Autodesk Fusion 360 part; units mm, degrees
(part 27 of 40)
  spline S73 degree 5 poles (31.1115, 52.5103) (31.1272, 52.5368) (31.1594, 52.5895) (31.2097, 52.6672) (31.2807, 52.7681) (31.3748, 52.8906) (31.4727, 53.0106) (31.5729, 53.1289) (31.6744, 53.2464) (31.7767, 53.3634) (31.88, 53.4797) (31.9844, 53.5951) (32.0903, 53.7094) (32.1981, 53.8224) (32.3077, 53.934) (32.419, 54.0444) (32.5316, 54.1537) (32.6455, 54.2622) (32.7603, 54.3698) (32.876, 54.4767) (32.9927, 54.5828) (33.1105, 54.6881) (33.2292, 54.7926) (33.3491, 54.8961) (33.47, 54.9988) (33.5919, 55.1007) (33.7148, 55.2017) (33.8386, 55.302) (33.9633, 55.4015) (34.0888, 55.5003) (34.2151, 55.5984) (34.3423, 55.6957) (34.4703, 55.7923) (34.5991, 55.8881) (34.7288, 55.9832) (34.8592, 56.0776) (34.9905, 56.1712) (35.1224, 56.2642) (35.2552, 56.3564) (35.3886, 56.448) (35.5228, 56.5388) (35.6577, 56.629) (35.7933, 56.7185) (35.9295, 56.8073) (36.0665, 56.8955) (36.2042, 56.9829) (36.3425, 57.0697) (36.4815, 57.1558) (36.6211, 57.2413) (36.7614, 57.3261) (36.9023, 57.4102) (37.0438, 57.4937) (37.186, 57.5765) (37.3288, 57.6587) (37.4721, 57.7403) (37.6161, 57.8212) (37.7607, 57.9014) (37.9058, 57.981) (38.0515, 58.06) (38.1978, 58.1383) (38.3447, 58.216) (38.4921, 58.2931) (38.6401, 58.3695) (38.7886, 58.4453) (38.9377, 58.5205) (39.0873, 58.595) (39.2374, 58.669) (39.3881, 58.7423) (39.5393, 58.8149) (39.6909, 58.887) (39.8431, 58.9584) (39.9653, 59.0151) (40.0572, 59.0573) (40.1185, 59.0853) (40.1492, 59.0993) knots 0 0 0 0 0 0 0.01428571 0.02857143 0.04285714 0.05714286 0.07142857 0.08571429 0.1 0.11428571 0.12857143 0.14285714 0.15714286 0.17142857 0.18571429 0.2 0.21428571 0.22857143 0.24285714 0.25714286 0.27142857 0.28571429 0.3 0.31428571 0.32857143 0.34285714 0.35714286 0.37142857 0.38571429 0.4 0.41428571 0.42857143 0.44285714 0.45714286 0.47142857 0.48571429 0.5 0.51428571 0.52857143 0.54285714 0.55714286 0.57142857 0.58571429 0.6 0.61428571 0.62857143 0.64285714 0.65714286 0.67142857 0.68571429 0.7 0.71428571 0.72857143 0.74285714 0.75714286 0.77142857 0.78571429 0.8 0.81428571 0.82857143 0.84285714 0.85714286 0.87142857 0.88571429 0.9 0.91428571 0.92857143 0.94285714 0.95714286 0.97142857 0.98571429 1 1 1 1 1 1
  line L5468 (31.1115, 52.5103) -> (31.1272, 52.5368) construction
  line L5469 (31.1272, 52.5368) -> (31.1594, 52.5895) construction
  line L5470 (31.1594, 52.5895) -> (31.2097, 52.6672) construction
  line L5471 (31.2097, 52.6672) -> (31.2807, 52.7681) construction
  line L5472 (31.2807, 52.7681) -> (31.3748, 52.8906) construction
  line L5473 (31.3748, 52.8906) -> (31.4727, 53.0106) construction
  line L5474 (31.4727, 53.0106) -> (31.5729, 53.1289) construction
  line L5475 (31.5729, 53.1289) -> (31.6744, 53.2464) construction
  line L5476 (31.6744, 53.2464) -> (31.7767, 53.3634) construction
  line L5477 (31.7767, 53.3634) -> (31.88, 53.4797) construction
  line L5478 (31.88, 53.4797) -> (31.9844, 53.5951) construction
  line L5479 (31.9844, 53.5951) -> (32.0903, 53.7094) construction
  line L5480 (32.0903, 53.7094) -> (32.1981, 53.8224) construction
  line L5481 (32.1981, 53.8224) -> (32.3077, 53.934) construction
  line L5482 (32.3077, 53.934) -> (32.419, 54.0444) construction
  line L5483 (32.419, 54.0444) -> (32.5316, 54.1537) construction
  line L5484 (32.5316, 54.1537) -> (32.6455, 54.2622) construction
  line L5485 (32.6455, 54.2622) -> (32.7603, 54.3698) construction
  line L5486 (32.7603, 54.3698) -> (32.876, 54.4767) construction
  line L5487 (32.876, 54.4767) -> (32.9927, 54.5828) construction
  line L5488 (32.9927, 54.5828) -> (33.1105, 54.6881) construction
  line L5489 (33.1105, 54.6881) -> (33.2292, 54.7926) construction
  line L5490 (33.2292, 54.7926) -> (33.3491, 54.8961) construction
  line L5491 (33.3491, 54.8961) -> (33.47, 54.9988) construction
  line L5492 (33.47, 54.9988) -> (33.5919, 55.1007) construction
  line L5493 (33.5919, 55.1007) -> (33.7148, 55.2017) construction
  line L5494 (33.7148, 55.2017) -> (33.8386, 55.302) construction
  line L5495 (33.8386, 55.302) -> (33.9633, 55.4015) construction
  line L5496 (33.9633, 55.4015) -> (34.0888, 55.5003) construction
  line L5497 (34.0888, 55.5003) -> (34.2151, 55.5984) construction
  line L5498 (34.2151, 55.5984) -> (34.3423, 55.6957) construction
  line L5499 (34.3423, 55.6957) -> (34.4703, 55.7923) construction
  line L5500 (34.4703, 55.7923) -> (34.5991, 55.8881) construction
  line L5501 (34.5991, 55.8881) -> (34.7288, 55.9832) construction
  line L5502 (34.7288, 55.9832) -> (34.8592, 56.0776) construction
  line L5503 (34.8592, 56.0776) -> (34.9905, 56.1712) construction
  line L5504 (34.9905, 56.1712) -> (35.1224, 56.2642) construction
  line L5505 (35.1224, 56.2642) -> (35.2552, 56.3564) construction
  line L5506 (35.2552, 56.3564) -> (35.3886, 56.448) construction
  line L5507 (35.3886, 56.448) -> (35.5228, 56.5388) construction
  line L5508 (35.5228, 56.5388) -> (35.6577, 56.629) construction
  line L5509 (35.6577, 56.629) -> (35.7933, 56.7185) construction
  line L5510 (35.7933, 56.7185) -> (35.9295, 56.8073) construction
  line L5511 (35.9295, 56.8073) -> (36.0665, 56.8955) construction
  line L5512 (36.0665, 56.8955) -> (36.2042, 56.9829) construction
  line L5513 (36.2042, 56.9829) -> (36.3425, 57.0697) construction
  line L5514 (36.3425, 57.0697) -> (36.4815, 57.1558) construction
  line L5515 (36.4815, 57.1558) -> (36.6211, 57.2413) construction
  line L5516 (36.6211, 57.2413) -> (36.7614, 57.3261) construction
  line L5517 (36.7614, 57.3261) -> (36.9023, 57.4102) construction
  line L5518 (36.9023, 57.4102) -> (37.0438, 57.4937) construction
  line L5519 (37.0438, 57.4937) -> (37.186, 57.5765) construction
  line L5520 (37.186, 57.5765) -> (37.3288, 57.6587) construction
  line L5521 (37.3288, 57.6587) -> (37.4721, 57.7403) construction
  line L5522 (37.4721, 57.7403) -> (37.6161, 57.8212) construction
  line L5523 (37.6161, 57.8212) -> (37.7607, 57.9014) construction
  line L5524 (37.7607, 57.9014) -> (37.9058, 57.981) construction
  line L5525 (37.9058, 57.981) -> (38.0515, 58.06) construction
  line L5526 (38.0515, 58.06) -> (38.1978, 58.1383) construction
  line L5527 (38.1978, 58.1383) -> (38.3447, 58.216) construction
  line L5528 (38.3447, 58.216) -> (38.4921, 58.2931) construction
  line L5529 (38.4921, 58.2931) -> (38.6401, 58.3695) construction
  line L5530 (38.6401, 58.3695) -> (38.7886, 58.4453) construction
  line L5531 (38.7886, 58.4453) -> (38.9377, 58.5205) construction
  line L5532 (38.9377, 58.5205) -> (39.0873, 58.595) construction
  line L5533 (39.0873, 58.595) -> (39.2374, 58.669) construction
  line L5534 (39.2374, 58.669) -> (39.3881, 58.7423) construction
  line L5535 (39.3881, 58.7423) -> (39.5393, 58.8149) construction
  line L5536 (39.5393, 58.8149) -> (39.6909, 58.887) construction
  line L5537 (39.6909, 58.887) -> (39.8431, 58.9584) construction
  line L5538 (39.8431, 58.9584) -> (39.9653, 59.0151) construction
  line L5539 (39.9653, 59.0151) -> (40.0572, 59.0573) construction
  line L5540 (40.0572, 59.0573) -> (40.1185, 59.0853) construction
  line L5541 (40.1185, 59.0853) -> (40.1492, 59.0993) construction
  arc A139 (51.9354, 24.5301) -> (54.5366, 23.5481) centre (53.7438, 25.3842) ccw
  spline S74 degree 5 poles (52.5103, -31.1115) (52.5368, -31.1272) (52.5895, -31.1594) (52.6672, -31.2097) (52.7681, -31.2807) (52.8906, -31.3748) (53.0106, -31.4727) (53.1289, -31.5729) (53.2464, -31.6744) (53.3634, -31.7767) (53.4797, -31.88) (53.5951, -31.9844) (53.7094, -32.0903) (53.8224, -32.1981) (53.934, -32.3077) (54.0444, -32.419) (54.1537, -32.5316) (54.2622, -32.6455) (54.3698, -32.7603) (54.4767, -32.876) (54.5828, -32.9927) (54.6881, -33.1105) (54.7926, -33.2292) (54.8961, -33.3491) (54.9988, -33.47) (55.1007, -33.5919) (55.2017, -33.7148) (55.302, -33.8386) (55.4015, -33.9633) (55.5003, -34.0888) (55.5984, -34.2151) (55.6957, -34.3423) (55.7923, -34.4703) (55.8881, -34.5991) (55.9832, -34.7288) (56.0776, -34.8592) (56.1712, -34.9905) (56.2642, -35.1224) (56.3564, -35.2552) (56.448, -35.3886) (56.5388, -35.5228) (56.629, -35.6577) (56.7185, -35.7933) (56.8073, -35.9295) (56.8955, -36.0665) (56.9829, -36.2042) (57.0697, -36.3425) (57.1558, -36.4815) (57.2413, -36.6211) (57.3261, -36.7614) (57.4102, -36.9023) (57.4937, -37.0438) (57.5765, -37.186) (57.6587, -37.3288) (57.7403, -37.4721) (57.8212, -37.6161) (57.9014, -37.7607) (57.981, -37.9058) (58.06, -38.0515) (58.1383, -38.1978) (58.216, -38.3447) (58.2931, -38.4921) (58.3695, -38.6401) (58.4453, -38.7886) (58.5205, -38.9377) (58.595, -39.0873) (58.669, -39.2374) (58.7423, -39.3881) (58.8149, -39.5393) (58.887, -39.6909) (58.9584, -39.8431) (59.0151, -39.9653) (59.0573, -40.0572) (59.0853, -40.1185) (59.0993, -40.1492) knots 0 0 0 0 0 0 0.01428571 0.02857143 0.04285714 0.05714286 0.07142857 0.08571429 0.1 0.11428571 0.12857143 0.14285714 0.15714286 0.17142857 0.18571429 0.2 0.21428571 0.22857143 0.24285714 0.25714286 0.27142857 0.28571429 0.3 0.31428571 0.32857143 0.34285714 0.35714286 0.37142857 0.38571429 0.4 0.41428571 0.42857143 0.44285714 0.45714286 0.47142857 0.48571429 0.5 0.51428571 0.52857143 0.54285714 0.55714286 0.57142857 0.58571429 0.6 0.61428571 0.62857143 0.64285714 0.65714286 0.67142857 0.68571429 0.7 0.71428571 0.72857143 0.74285714 0.75714286 0.77142857 0.78571429 0.8 0.81428571 0.82857143 0.84285714 0.85714286 0.87142857 0.88571429 0.9 0.91428571 0.92857143 0.94285714 0.95714286 0.97142857 0.98571429 1 1 1 1 1 1
  line L5542 (52.5103, -31.1115) -> (52.5368, -31.1272) construction
  line L5543 (52.5368, -31.1272) -> (52.5895, -31.1594) construction
  line L5544 (52.5895, -31.1594) -> (52.6672, -31.2097) construction
  line L5545 (52.6672, -31.2097) -> (52.7681, -31.2807) construction
  line L5546 (52.7681, -31.2807) -> (52.8906, -31.3748) construction
  line L5547 (52.8906, -31.3748) -> (53.0106, -31.4727) construction
  line L5548 (53.0106, -31.4727) -> (53.1289, -31.5729) construction
  line L5549 (53.1289, -31.5729) -> (53.2464, -31.6744) construction
  line L5550 (53.2464, -31.6744) -> (53.3634, -31.7767) construction
  line L5551 (53.3634, -31.7767) -> (53.4797, -31.88) construction
  line L5552 (53.4797, -31.88) -> (53.5951, -31.9844) construction
  line L5553 (53.5951, -31.9844) -> (53.7094, -32.0903) construction
  line L5554 (53.7094, -32.0903) -> (53.8224, -32.1981) construction
  line L5555 (53.8224, -32.1981) -> (53.934, -32.3077) construction
  line L5556 (53.934, -32.3077) -> (54.0444, -32.419) construction
  line L5557 (54.0444, -32.419) -> (54.1537, -32.5316) construction
  line L5558 (54.1537, -32.5316) -> (54.2622, -32.6455) construction
  line L5559 (54.2622, -32.6455) -> (54.3698, -32.7603) construction
  line L5560 (54.3698, -32.7603) -> (54.4767, -32.876) construction
  line L5561 (54.4767, -32.876) -> (54.5828, -32.9927) construction
  line L5562 (54.5828, -32.9927) -> (54.6881, -33.1105) construction
  line L5563 (54.6881, -33.1105) -> (54.7926, -33.2292) construction
  line L5564 (54.7926, -33.2292) -> (54.8961, -33.3491) construction
  line L5565 (54.8961, -33.3491) -> (54.9988, -33.47) construction
  line L5566 (54.9988, -33.47) -> (55.1007, -33.5919) construction
  line L5567 (55.1007, -33.5919) -> (55.2017, -33.7148) construction
  line L5568 (55.2017, -33.7148) -> (55.302, -33.8386) construction
  line L5569 (55.302, -33.8386) -> (55.4015, -33.9633) construction
  line L5570 (55.4015, -33.9633) -> (55.5003, -34.0888) construction
  line L5571 (55.5003, -34.0888) -> (55.5984, -34.2151) construction
  line L5572 (55.5984, -34.2151) -> (55.6957, -34.3423) construction
  line L5573 (55.6957, -34.3423) -> (55.7923, -34.4703) construction
  line L5574 (55.7923, -34.4703) -> (55.8881, -34.5991) construction
  line L5575 (55.8881, -34.5991) -> (55.9832, -34.7288) construction
  line L5576 (55.9832, -34.7288) -> (56.0776, -34.8592) construction
  line L5577 (56.0776, -34.8592) -> (56.1712, -34.9905) construction
  line L5578 (56.1712, -34.9905) -> (56.2642, -35.1224) construction
  line L5579 (56.2642, -35.1224) -> (56.3564, -35.2552) construction
  line L5580 (56.3564, -35.2552) -> (56.448, -35.3886) construction
  line L5581 (56.448, -35.3886) -> (56.5388, -35.5228) construction
  line L5582 (56.5388, -35.5228) -> (56.629, -35.6577) construction
  line L5583 (56.629, -35.6577) -> (56.7185, -35.7933) construction
  line L5584 (56.7185, -35.7933) -> (56.8073, -35.9295) construction
  line L5585 (56.8073, -35.9295) -> (56.8955, -36.0665) construction
  line L5586 (56.8955, -36.0665) -> (56.9829, -36.2042) construction
  line L5587 (56.9829, -36.2042) -> (57.0697, -36.3425) construction
  line L5588 (57.0697, -36.3425) -> (57.1558, -36.4815) construction
  line L5589 (57.1558, -36.4815) -> (57.2413, -36.6211) construction
  line L5590 (57.2413, -36.6211) -> (57.3261, -36.7614) construction
  line L5591 (57.3261, -36.7614) -> (57.4102, -36.9023) construction
  line L5592 (57.4102, -36.9023) -> (57.4937, -37.0438) construction
  line L5593 (57.4937, -37.0438) -> (57.5765, -37.186) construction
  line L5594 (57.5765, -37.186) -> (57.6587, -37.3288) construction
  line L5595 (57.6587, -37.3288) -> (57.7403, -37.4721) construction
  line L5596 (57.7403, -37.4721) -> (57.8212, -37.6161) construction
  line L5597 (57.8212, -37.6161) -> (57.9014, -37.7607) construction
  line L5598 (57.9014, -37.7607) -> (57.981, -37.9058) construction
  line L5599 (57.981, -37.9058) -> (58.06, -38.0515) construction
  line L5600 (58.06, -38.0515) -> (58.1383, -38.1978) construction
  line L5601 (58.1383, -38.1978) -> (58.216, -38.3447) construction
  line L5602 (58.216, -38.3447) -> (58.2931, -38.4921) construction
  line L5603 (58.2931, -38.4921) -> (58.3695, -38.6401) construction
  line L5604 (58.3695, -38.6401) -> (58.4453, -38.7886) construction
  line L5605 (58.4453, -38.7886) -> (58.5205, -38.9377) construction
  line L5606 (58.5205, -38.9377) -> (58.595, -39.0873) construction
  line L5607 (58.595, -39.0873) -> (58.669, -39.2374) construction
  line L5608 (58.669, -39.2374) -> (58.7423, -39.3881) construction
  line L5609 (58.7423, -39.3881) -> (58.8149, -39.5393) construction
  line L5610 (58.8149, -39.5393) -> (58.887, -39.6909) construction
  line L5611 (58.887, -39.6909) -> (58.9584, -39.8431) construction
  line L5612 (58.9584, -39.8431) -> (59.0151, -39.9653) construction
  line L5613 (59.0151, -39.9653) -> (59.0573, -40.0572) construction
  line L5614 (59.0573, -40.0572) -> (59.0853, -40.1185) construction
  line L5615 (59.0853, -40.1185) -> (59.0993, -40.1492) construction
  arc A140 (59.0993, 40.1492) -> (56.4469, 43.8) centre (0, 0) ccw
  line L5616 (-23.5481, -54.5366) -> (-24.1948, -56.0345)
  line L5617 (44.5906, -39.2483) -> (45.8153, -40.3263)
  line L5618 (-44.5906, -39.2483) -> (-45.8153, -40.3263)
  arc A141 (23.5481, 54.5366) -> (24.5301, 51.9354) centre (25.3842, 53.7438) ccw
  arc A142 (39.2483, 44.5906) -> (39.3784, 41.8132) centre (40.7496, 43.2692) ccw
  arc A143 (5.5428, 59.1442) -> (7.2806, 56.9737) centre (7.5341, 58.9575) ccw
  arc A144 (13.005, -57.9623) -> (10.6816, -56.435) centre (11.0535, -58.4001) ccw
  spline S75 degree 5 poles (-24.1948, -56.0345) (-24.2071, -56.0628) (-24.2308, -56.1198) (-24.264, -56.2062) (-24.3039, -56.3229) (-24.3478, -56.4711) (-24.3873, -56.6208) (-24.4241, -56.7714) (-24.4595, -56.9226) (-24.494, -57.0741) (-24.5274, -57.226) (-24.5594, -57.3783) (-24.5896, -57.5312) (-24.6176, -57.6848) (-24.6435, -57.8391) (-24.6674, -57.994) (-24.6897, -58.1494) (-24.7105, -58.3052) (-24.7301, -58.4614) (-24.7485, -58.6179) (-24.7658, -58.7747) (-24.7818, -58.9318) (-24.7965, -59.0893) (-24.8098, -59.2471) (-24.8218, -59.4053) (-24.8325, -59.5638) (-24.842, -59.7226) (-24.8504, -59.8817) (-24.8577, -60.0411) (-24.8638, -60.2007) (-24.8689, -60.3605) (-24.8729, -60.5206) (-24.8757, -60.6809) (-24.8776, -60.8415) (-24.8783, -61.0023) (-24.878, -61.1633) (-24.8766, -61.3245) (-24.8742, -61.4859) (-24.8708, -61.6475) (-24.8665, -61.8093) (-24.8611, -61.9712) (-24.8548, -62.1334) (-24.8475, -62.2957) (-24.8392, -62.4581) (-24.83, -62.6207) (-24.8199, -62.7835) (-24.8088, -62.9464) (-24.7967, -63.1095) (-24.7838, -63.2727) (-24.77, -63.436) (-24.7552, -63.5995) (-24.7396, -63.7631) (-24.723, -63.9268) (-24.7056, -64.0906) (-24.6873, -64.2545) (-24.6681, -64.4185) (-24.648, -64.5826) (-24.6271, -64.7468) (-24.6054, -64.9111) (-24.5828, -65.0755) (-24.5593, -65.24) (-24.535, -65.4046) (-24.5098, -65.5692) (-24.4839, -65.734) (-24.4571, -65.8987) (-24.4294, -66.0636) (-24.401, -66.2285) (-24.3718, -66.3935) (-24.3417, -66.5585) (-24.3108, -66.7236) (-24.2792, -66.8887) (-24.2532, -67.0208) (-24.2334, -67.1199) (-24.22, -67.186) (-24.2132, -67.2191) knots 0 0 0 0 0 0 0.01428571 0.02857143 0.04285714 0.05714286 0.07142857 0.08571429 0.1 0.11428571 0.12857143 0.14285714 0.15714286 0.17142857 0.18571429 0.2 0.21428571 0.22857143 0.24285714 0.25714286 0.27142857 0.28571429 0.3 0.31428571 0.32857143 0.34285714 0.35714286 0.37142857 0.38571429 0.4 0.41428571 0.42857143 0.44285714 0.45714286 0.47142857 0.48571429 0.5 0.51428571 0.52857143 0.54285714 0.55714286 0.57142857 0.58571429 0.6 0.61428571 0.62857143 0.64285714 0.65714286 0.67142857 0.68571429 0.7 0.71428571 0.72857143 0.74285714 0.75714286 0.77142857 0.78571429 0.8 0.81428571 0.82857143 0.84285714 0.85714286 0.87142857 0.88571429 0.9 0.91428571 0.92857143 0.94285714 0.95714286 0.97142857 0.98571429 1 1 1 1 1 1
  line L5619 (-24.1948, -56.0345) -> (-24.2071, -56.0628) construction
  line L5620 (-24.2071, -56.0628) -> (-24.2308, -56.1198) construction
  line L5621 (-24.2308, -56.1198) -> (-24.264, -56.2062) construction
  line L5622 (-24.264, -56.2062) -> (-24.3039, -56.3229) construction
  line L5623 (-24.3039, -56.3229) -> (-24.3478, -56.4711) construction
  line L5624 (-24.3478, -56.4711) -> (-24.3873, -56.6208) construction
  line L5625 (-24.3873, -56.6208) -> (-24.4241, -56.7714) construction
  line L5626 (-24.4241, -56.7714) -> (-24.4595, -56.9226) construction
  line L5627 (-24.4595, -56.9226) -> (-24.494, -57.0741) construction
  line L5628 (-24.494, -57.0741) -> (-24.5274, -57.226) construction
  line L5629 (-24.5274, -57.226) -> (-24.5594, -57.3783) construction
  line L5630 (-24.5594, -57.3783) -> (-24.5896, -57.5312) construction
  line L5631 (-24.5896, -57.5312) -> (-24.6176, -57.6848) construction
  line L5632 (-24.6176, -57.6848) -> (-24.6435, -57.8391) construction
  line L5633 (-24.6435, -57.8391) -> (-24.6674, -57.994) construction
  line L5634 (-24.6674, -57.994) -> (-24.6897, -58.1494) construction
  line L5635 (-24.6897, -58.1494) -> (-24.7105, -58.3052) construction
  line L5636 (-24.7105, -58.3052) -> (-24.7301, -58.4614) construction
  line L5637 (-24.7301, -58.4614) -> (-24.7485, -58.6179) construction
  line L5638 (-24.7485, -58.6179) -> (-24.7658, -58.7747) construction
  line L5639 (-24.7658, -58.7747) -> (-24.7818, -58.9318) construction
  line L5640 (-24.7818, -58.9318) -> (-24.7965, -59.0893) construction
  line L5641 (-24.7965, -59.0893) -> (-24.8098, -59.2471) construction
  line L5642 (-24.8098, -59.2471) -> (-24.8218, -59.4053) construction
  line L5643 (-24.8218, -59.4053) -> (-24.8325, -59.5638) construction
  line L5644 (-24.8325, -59.5638) -> (-24.842, -59.7226) construction
  line L5645 (-24.842, -59.7226) -> (-24.8504, -59.8817) construction
  line L5646 (-24.8504, -59.8817) -> (-24.8577, -60.0411) construction
  line L5647 (-24.8577, -60.0411) -> (-24.8638, -60.2007) construction
  line L5648 (-24.8638, -60.2007) -> (-24.8689, -60.3605) construction
  line L5649 (-24.8689, -60.3605) -> (-24.8729, -60.5206) construction
  line L5650 (-24.8729, -60.5206) -> (-24.8757, -60.6809) construction
  line L5651 (-24.8757, -60.6809) -> (-24.8776, -60.8415) construction
  line L5652 (-24.8776, -60.8415) -> (-24.8783, -61.0023) construction
  line L5653 (-24.8783, -61.0023) -> (-24.878, -61.1633) construction
  line L5654 (-24.878, -61.1633) -> (-24.8766, -61.3245) construction
  line L5655 (-24.8766, -61.3245) -> (-24.8742, -61.4859) construction
  line L5656 (-24.8742, -61.4859) -> (-24.8708, -61.6475) construction
  line L5657 (-24.8708, -61.6475) -> (-24.8665, -61.8093) construction
  line L5658 (-24.8665, -61.8093) -> (-24.8611, -61.9712) construction
  line L5659 (-24.8611, -61.9712) -> (-24.8548, -62.1334) construction
  line L5660 (-24.8548, -62.1334) -> (-24.8475, -62.2957) construction
  line L5661 (-24.8475, -62.2957) -> (-24.8392, -62.4581) construction
  line L5662 (-24.8392, -62.4581) -> (-24.83, -62.6207) construction
  line L5663 (-24.83, -62.6207) -> (-24.8199, -62.7835) construction
  line L5664 (-24.8199, -62.7835) -> (-24.8088, -62.9464) construction
  line L5665 (-24.8088, -62.9464) -> (-24.7967, -63.1095) construction
  line L5666 (-24.7967, -63.1095) -> (-24.7838, -63.2727) construction
  line L5667 (-24.7838, -63.2727) -> (-24.77, -63.436) construction
  line L5668 (-24.77, -63.436) -> (-24.7552, -63.5995) construction
  line L5669 (-24.7552, -63.5995) -> (-24.7396, -63.7631) construction
  line L5670 (-24.7396, -63.7631) -> (-24.723, -63.9268) construction
  line L5671 (-24.723, -63.9268) -> (-24.7056, -64.0906) construction
  line L5672 (-24.7056, -64.0906) -> (-24.6873, -64.2545) construction
  line L5673 (-24.6873, -64.2545) -> (-24.6681, -64.4185) construction
  line L5674 (-24.6681, -64.4185) -> (-24.648, -64.5826) construction
  line L5675 (-24.648, -64.5826) -> (-24.6271, -64.7468) construction
  line L5676 (-24.6271, -64.7468) -> (-24.6054, -64.9111) construction
  line L5677 (-24.6054, -64.9111) -> (-24.5828, -65.0755) construction
  line L5678 (-24.5828, -65.0755) -> (-24.5593, -65.24) construction
  line L5679 (-24.5593, -65.24) -> (-24.535, -65.4046) construction
  line L5680 (-24.535, -65.4046) -> (-24.5098, -65.5692) construction
  line L5681 (-24.5098, -65.5692) -> (-24.4839, -65.734) construction
  line L5682 (-24.4839, -65.734) -> (-24.4571, -65.8987) construction
  line L5683 (-24.4571, -65.8987) -> (-24.4294, -66.0636) construction
  line L5684 (-24.4294, -66.0636) -> (-24.401, -66.2285) construction
  line L5685 (-24.401, -66.2285) -> (-24.3718, -66.3935) construction
  line L5686 (-24.3718, -66.3935) -> (-24.3417, -66.5585) construction
  line L5687 (-24.3417, -66.5585) -> (-24.3108, -66.7236) construction
  line L5688 (-24.3108, -66.7236) -> (-24.2792, -66.8887) construction
  line L5689 (-24.2792, -66.8887) -> (-24.2532, -67.0208) construction
  line L5690 (-24.2532, -67.0208) -> (-24.2334, -67.1199) construction
  line L5691 (-24.2334, -67.1199) -> (-24.22, -67.186) construction
  line L5692 (-24.22, -67.186) -> (-24.2132, -67.2191) construction
  arc A145 (56.435, -10.6816) -> (57.9623, -13.005) centre (58.4001, -11.0535) ccw
  arc A146 (-24.2132, -67.2191) -> (-19.9215, -68.6136) centre (0, 0) ccw
  arc A147 (-71.4115, 2.2563) -> (-71.4115, -2.2563) centre (0, 0) ccw
  arc A148 (30.2798, -51.1066) -> (27.5982, -50.3721) centre (28.5592, -52.1261) ccw
  spline S76 degree 5 poles (-60.7685, 5.6951) (-60.7993, 5.6979) (-60.8609, 5.7029) (-60.9533, 5.7078) (-61.0766, 5.7097) (-61.231, 5.7056) (-61.3856, 5.6969) (-61.5403, 5.6854) (-61.695, 5.6723) (-61.8498, 5.6583) (-62.0045, 5.6431) (-62.1593, 5.6265) (-62.314, 5.608) (-62.4688, 5.5871) (-62.6235, 5.5641) (-62.7782, 5.539) (-62.9329, 5.5121) (-63.0875, 5.4838) (-63.2421, 5.4542) (-63.3966, 5.4233) (-63.5511, 5.3913) (-63.7055, 5.3579) (-63.8598, 5.3232) (-64.014, 5.2871) (-64.1682, 5.2497) (-64.3222, 5.2109) (-64.4762, 5.1709) (-64.6301, 5.1297) (-64.7839, 5.0873) (-64.9376, 5.0439) (-65.0912, 4.9993) (-65.2447, 4.9536) (-65.398, 4.9068) (-65.5513, 4.8589) (-65.7044, 4.8099) (-65.8574, 4.7599) (-66.0103, 4.7087) (-66.1631, 4.6566) (-66.3158, 4.6035) (-66.4683, 4.5493) (-66.6206, 4.4942) (-66.7729, 4.438) (-66.925, 4.381) (-67.077, 4.3229) (-67.2288, 4.2639) (-67.3804, 4.2039) (-67.532, 4.143) (-67.6833, 4.0812) (-67.8345, 4.0185) (-67.9856, 3.9548) (-68.1365, 3.8903) (-68.2872, 3.8249) (-68.4378, 3.7585) (-68.5882, 3.6913) (-68.7384, 3.6233) (-68.8885, 3.5543) (-69.0384, 3.4846) (-69.1881, 3.4139) (-69.3376, 3.3425) (-69.487, 3.2701) (-69.6362, 3.197) (-69.7852, 3.123) (-69.934, 3.0482) (-70.0826, 2.9726) (-70.2311, 2.8962) (-70.3793, 2.819) (-70.5274, 2.741) (-70.6752, 2.6622) (-70.8229, 2.5826) (-70.9703, 2.5023) (-71.1176, 2.4211) (-71.2352, 2.3556) (-71.3234, 2.3061) (-71.3821, 2.2729) (-71.4115, 2.2563) knots 0 0 0 0 0 0 0.01428571 0.02857143 0.04285714 0.05714286 0.07142857 0.08571429 0.1 0.11428571 0.12857143 0.14285714 0.15714286 0.17142857 0.18571429 0.2 0.21428571 0.22857143 0.24285714 0.25714286 0.27142857 0.28571429 0.3 0.31428571 0.32857143 0.34285714 0.35714286 0.37142857 0.38571429 0.4 0.41428571 0.42857143 0.44285714 0.45714286 0.47142857 0.48571429 0.5 0.51428571 0.52857143 0.54285714 0.55714286 0.57142857 0.58571429 0.6 0.61428571 0.62857143 0.64285714 0.65714286 0.67142857 0.68571429 0.7 0.71428571 0.72857143 0.74285714 0.75714286 0.77142857 0.78571429 0.8 0.81428571 0.82857143 0.84285714 0.85714286 0.87142857 0.88571429 0.9 0.91428571 0.92857143 0.94285714 0.95714286 0.97142857 0.98571429 1 1 1 1 1 1
  line L5693 (-60.7685, 5.6951) -> (-60.7993, 5.6979) construction
  line L5694 (-60.7993, 5.6979) -> (-60.8609, 5.7029) construction
  line L5695 (-60.8609, 5.7029) -> (-60.9533, 5.7078) construction
  line L5696 (-60.9533, 5.7078) -> (-61.0766, 5.7097) construction
  line L5697 (-61.0766, 5.7097) -> (-61.231, 5.7056) construction
  line L5698 (-61.231, 5.7056) -> (-61.3856, 5.6969) construction
  line L5699 (-61.3856, 5.6969) -> (-61.5403, 5.6854) construction
  line L5700 (-61.5403, 5.6854) -> (-61.695, 5.6723) construction
  line L5701 (-61.695, 5.6723) -> (-61.8498, 5.6583) construction
  line L5702 (-61.8498, 5.6583) -> (-62.0045, 5.6431) construction
  line L5703 (-62.0045, 5.6431) -> (-62.1593, 5.6265) construction
  line L5704 (-62.1593, 5.6265) -> (-62.314, 5.608) construction
  line L5705 (-62.314, 5.608) -> (-62.4688, 5.5871) construction
  line L5706 (-62.4688, 5.5871) -> (-62.6235, 5.5641) construction
  line L5707 (-62.6235, 5.5641) -> (-62.7782, 5.539) construction
  line L5708 (-62.7782, 5.539) -> (-62.9329, 5.5121) construction
  line L5709 (-62.9329, 5.5121) -> (-63.0875, 5.4838) construction
  line L5710 (-63.0875, 5.4838) -> (-63.2421, 5.4542) construction
  line L5711 (-63.2421, 5.4542) -> (-63.3966, 5.4233) construction
  line L5712 (-63.3966, 5.4233) -> (-63.5511, 5.3913) construction
  line L5713 (-63.5511, 5.3913) -> (-63.7055, 5.3579) construction
  line L5714 (-63.7055, 5.3579) -> (-63.8598, 5.3232) construction
  line L5715 (-63.8598, 5.3232) -> (-64.014, 5.2871) construction
  line L5716 (-64.014, 5.2871) -> (-64.1682, 5.2497) construction
  line L5717 (-64.1682, 5.2497) -> (-64.3222, 5.2109) construction
  line L5718 (-64.3222, 5.2109) -> (-64.4762, 5.1709) construction
  line L5719 (-64.4762, 5.1709) -> (-64.6301, 5.1297) construction
  line L5720 (-64.6301, 5.1297) -> (-64.7839, 5.0873) construction
  line L5721 (-64.7839, 5.0873) -> (-64.9376, 5.0439) construction
  line L5722 (-64.9376, 5.0439) -> (-65.0912, 4.9993) construction
  line L5723 (-65.0912, 4.9993) -> (-65.2447, 4.9536) construction
  line L5724 (-65.2447, 4.9536) -> (-65.398, 4.9068) construction
  line L5725 (-65.398, 4.9068) -> (-65.5513, 4.8589) construction
  line L5726 (-65.5513, 4.8589) -> (-65.7044, 4.8099) construction
  line L5727 (-65.7044, 4.8099) -> (-65.8574, 4.7599) construction
  line L5728 (-65.8574, 4.7599) -> (-66.0103, 4.7087) construction
  line L5729 (-66.0103, 4.7087) -> (-66.1631, 4.6566) construction
  line L5730 (-66.1631, 4.6566) -> (-66.3158, 4.6035) construction
  line L5731 (-66.3158, 4.6035) -> (-66.4683, 4.5493) construction
  line L5732 (-66.4683, 4.5493) -> (-66.6206, 4.4942) construction
  line L5733 (-66.6206, 4.4942) -> (-66.7729, 4.438) construction
  line L5734 (-66.7729, 4.438) -> (-66.925, 4.381) construction
  line L5735 (-66.925, 4.381) -> (-67.077, 4.3229) construction
  line L5736 (-67.077, 4.3229) -> (-67.2288, 4.2639) construction
  line L5737 (-67.2288, 4.2639) -> (-67.3804, 4.2039) construction
  line L5738 (-67.3804, 4.2039) -> (-67.532, 4.143) construction
  line L5739 (-67.532, 4.143) -> (-67.6833, 4.0812) construction
  line L5740 (-67.6833, 4.0812) -> (-67.8345, 4.0185) construction
  line L5741 (-67.8345, 4.0185) -> (-67.9856, 3.9548) construction
  line L5742 (-67.9856, 3.9548) -> (-68.1365, 3.8903) construction
  line L5743 (-68.1365, 3.8903) -> (-68.2872, 3.8249) construction
  line L5744 (-68.2872, 3.8249) -> (-68.4378, 3.7585) construction
  line L5745 (-68.4378, 3.7585) -> (-68.5882, 3.6913) construction
  line L5746 (-68.5882, 3.6913) -> (-68.7384, 3.6233) construction
  line L5747 (-68.7384, 3.6233) -> (-68.8885, 3.5543) construction
  line L5748 (-68.8885, 3.5543) -> (-69.0384, 3.4846) construction
  line L5749 (-69.0384, 3.4846) -> (-69.1881, 3.4139) construction
  line L5750 (-69.1881, 3.4139) -> (-69.3376, 3.3425) construction
  line L5751 (-69.3376, 3.3425) -> (-69.487, 3.2701) construction
  line L5752 (-69.487, 3.2701) -> (-69.6362, 3.197) construction
  line L5753 (-69.6362, 3.197) -> (-69.7852, 3.123) construction
  line L5754 (-69.7852, 3.123) -> (-69.934, 3.0482) construction
  line L5755 (-69.934, 3.0482) -> (-70.0826, 2.9726) construction
  line L5756 (-70.0826, 2.9726) -> (-70.2311, 2.8962) construction
  line L5757 (-70.2311, 2.8962) -> (-70.3793, 2.819) construction
  line L5758 (-70.3793, 2.819) -> (-70.5274, 2.741) construction
  line L5759 (-70.5274, 2.741) -> (-70.6752, 2.6622) construction
  line L5760 (-70.6752, 2.6622) -> (-70.8229, 2.5826) construction
  line L5761 (-70.8229, 2.5826) -> (-70.9703, 2.5023) construction
  line L5762 (-70.9703, 2.5023) -> (-71.1176, 2.4211) construction
  line L5763 (-71.1176, 2.4211) -> (-71.2352, 2.3556) construction
  line L5764 (-71.2352, 2.3556) -> (-71.3234, 2.3061) construction
  line L5765 (-71.3234, 2.3061) -> (-71.3821, 2.2729) construction
  line L5766 (-71.3821, 2.2729) -> (-71.4115, 2.2563) construction
  spline S77 degree 5 poles (56.0345, 24.1948) (56.0628, 24.2071) (56.1198, 24.2308) (56.2062, 24.264) (56.3229, 24.3039) (56.4711, 24.3478) (56.6208, 24.3873) (56.7714, 24.4241) (56.9226, 24.4595) (57.0741, 24.494) (57.226, 24.5274) (57.3783, 24.5594) (57.5312, 24.5896) (57.6848, 24.6176) (57.8391, 24.6435) (57.994, 24.6674) (58.1494, 24.6897) (58.3052, 24.7105) (58.4614, 24.7301) (58.6179, 24.7485) (58.7747, 24.7658) (58.9318, 24.7818) (59.0893, 24.7965) (59.2471, 24.8098) (59.4053, 24.8218) (59.5638, 24.8325) (59.7226, 24.842) (59.8817, 24.8504) (60.0411, 24.8577) (60.2007, 24.8638) (60.3605, 24.8689) (60.5206, 24.8729) (60.6809, 24.8757) (60.8415, 24.8776) (61.0023, 24.8783) (61.1633, 24.878) (61.3245, 24.8766) (61.4859, 24.8742) (61.6475, 24.8708) (61.8093, 24.8665) (61.9712, 24.8611) (62.1334, 24.8548) (62.2957, 24.8475) (62.4581, 24.8392) (62.6207, 24.83) (62.7835, 24.8199) (62.9464, 24.8088) (63.1095, 24.7967) (63.2727, 24.7838) (63.436, 24.77) (63.5995, 24.7552) (63.7631, 24.7396) (63.9268, 24.723) (64.0906, 24.7056) (64.2545, 24.6873) (64.4185, 24.6681) (64.5826, 24.648) (64.7468, 24.6271) (64.9111, 24.6054) (65.0755, 24.5828) (65.24, 24.5593) (65.4046, 24.535) (65.5692, 24.5098) (65.734, 24.4839) (65.8987, 24.4571) (66.0636, 24.4294) (66.2285, 24.401) (66.3935, 24.3718) (66.5585, 24.3417) (66.7236, 24.3108) (66.8887, 24.2792) (67.0208, 24.2532) (67.1199, 24.2334) (67.186, 24.22) (67.2191, 24.2132) knots 0 0 0 0 0 0 0.01428571 0.02857143 0.04285714 0.05714286 0.07142857 0.08571429 0.1 0.11428571 0.12857143 0.14285714 0.15714286 0.17142857 0.18571429 0.2 0.21428571 0.22857143 0.24285714 0.25714286 0.27142857 0.28571429 0.3 0.31428571 0.32857143 0.34285714 0.35714286 0.37142857 0.38571429 0.4 0.41428571 0.42857143 0.44285714 0.45714286 0.47142857 0.48571429 0.5 0.51428571 0.52857143 0.54285714 0.55714286 0.57142857 0.58571429 0.6 0.61428571 0.62857143 0.64285714 0.65714286 0.67142857 0.68571429 0.7 0.71428571 0.72857143 0.74285714 0.75714286 0.77142857 0.78571429 0.8 0.81428571 0.82857143 0.84285714 0.85714286 0.87142857 0.88571429 0.9 0.91428571 0.92857143 0.94285714 0.95714286 0.97142857 0.98571429 1 1 1 1 1 1
  line L5767 (56.0345, 24.1948) -> (56.0628, 24.2071) construction
  line L5768 (56.0628, 24.2071) -> (56.1198, 24.2308) construction
  line L5769 (56.1198, 24.2308) -> (56.2062, 24.264) construction
  line L5770 (56.2062, 24.264) -> (56.3229, 24.3039) construction
  line L5771 (56.3229, 24.3039) -> (56.4711, 24.3478) construction
  line L5772 (56.4711, 24.3478) -> (56.6208, 24.3873) construction
  line L5773 (56.6208, 24.3873) -> (56.7714, 24.4241) construction
  line L5774 (56.7714, 24.4241) -> (56.9226, 24.4595) construction
  line L5775 (56.9226, 24.4595) -> (57.0741, 24.494) construction
  line L5776 (57.0741, 24.494) -> (57.226, 24.5274) construction
  line L5777 (57.226, 24.5274) -> (57.3783, 24.5594) construction
  line L5778 (57.3783, 24.5594) -> (57.5312, 24.5896) construction
  line L5779 (57.5312, 24.5896) -> (57.6848, 24.6176) construction
  line L5780 (57.6848, 24.6176) -> (57.8391, 24.6435) construction
  line L5781 (57.8391, 24.6435) -> (57.994, 24.6674) construction
  line L5782 (57.994, 24.6674) -> (58.1494, 24.6897) construction
  line L5783 (58.1494, 24.6897) -> (58.3052, 24.7105) construction
  line L5784 (58.3052, 24.7105) -> (58.4614, 24.7301) construction
  line L5785 (58.4614, 24.7301) -> (58.6179, 24.7485) construction
  line L5786 (58.6179, 24.7485) -> (58.7747, 24.7658) construction
  line L5787 (58.7747, 24.7658) -> (58.9318, 24.7818) construction
  line L5788 (58.9318, 24.7818) -> (59.0893, 24.7965) construction
  line L5789 (59.0893, 24.7965) -> (59.2471, 24.8098) construction
  line L5790 (59.2471, 24.8098) -> (59.4053, 24.8218) construction
  line L5791 (59.4053, 24.8218) -> (59.5638, 24.8325) construction
  line L5792 (59.5638, 24.8325) -> (59.7226, 24.842) construction
  line L5793 (59.7226, 24.842) -> (59.8817, 24.8504) construction
  line L5794 (59.8817, 24.8504) -> (60.0411, 24.8577) construction
  line L5795 (60.0411, 24.8577) -> (60.2007, 24.8638) construction
  line L5796 (60.2007, 24.8638) -> (60.3605, 24.8689) construction
  line L5797 (60.3605, 24.8689) -> (60.5206, 24.8729) construction
  line L5798 (60.5206, 24.8729) -> (60.6809, 24.8757) construction
  line L5799 (60.6809, 24.8757) -> (60.8415, 24.8776) construction
  line L5800 (60.8415, 24.8776) -> (61.0023, 24.8783) construction
  line L5801 (61.0023, 24.8783) -> (61.1633, 24.878) construction
  line L5802 (61.1633, 24.878) -> (61.3245, 24.8766) construction
  line L5803 (61.3245, 24.8766) -> (61.4859, 24.8742) construction
  line L5804 (61.4859, 24.8742) -> (61.6475, 24.8708) construction
  line L5805 (61.6475, 24.8708) -> (61.8093, 24.8665) construction
  line L5806 (61.8093, 24.8665) -> (61.9712, 24.8611) construction
  line L5807 (61.9712, 24.8611) -> (62.1334, 24.8548) construction
  line L5808 (62.1334, 24.8548) -> (62.2957, 24.8475) construction
  line L5809 (62.2957, 24.8475) -> (62.4581, 24.8392) construction
  line L5810 (62.4581, 24.8392) -> (62.6207, 24.83) construction
  line L5811 (62.6207, 24.83) -> (62.7835, 24.8199) construction
  line L5812 (62.7835, 24.8199) -> (62.9464, 24.8088) construction
  line L5813 (62.9464, 24.8088) -> (63.1095, 24.7967) construction
  line L5814 (63.1095, 24.7967) -> (63.2727, 24.7838) construction
  line L5815 (63.2727, 24.7838) -> (63.436, 24.77) construction
  line L5816 (63.436, 24.77) -> (63.5995, 24.7552) construction
  line L5817 (63.5995, 24.7552) -> (63.7631, 24.7396) construction
  line L5818 (63.7631, 24.7396) -> (63.9268, 24.723) construction
  line L5819 (63.9268, 24.723) -> (64.0906, 24.7056) construction
  line L5820 (64.0906, 24.7056) -> (64.2545, 24.6873) construction
  line L5821 (64.2545, 24.6873) -> (64.4185, 24.6681) construction
  line L5822 (64.4185, 24.6681) -> (64.5826, 24.648) construction
  line L5823 (64.5826, 24.648) -> (64.7468, 24.6271) construction
  line L5824 (64.7468, 24.6271) -> (64.9111, 24.6054) construction
  line L5825 (64.9111, 24.6054) -> (65.0755, 24.5828) construction
  line L5826 (65.0755, 24.5828) -> (65.24, 24.5593) construction
  line L5827 (65.24, 24.5593) -> (65.4046, 24.535) construction
  line L5828 (65.4046, 24.535) -> (65.5692, 24.5098) construction
  line L5829 (65.5692, 24.5098) -> (65.734, 24.4839) construction
  line L5830 (65.734, 24.4839) -> (65.8987, 24.4571) construction
  line L5831 (65.8987, 24.4571) -> (66.0636, 24.4294) construction
  line L5832 (66.0636, 24.4294) -> (66.2285, 24.401) construction
  line L5833 (66.2285, 24.401) -> (66.3935, 24.3718) construction
  line L5834 (66.3935, 24.3718) -> (66.5585, 24.3417) construction
  line L5835 (66.5585, 24.3417) -> (66.7236, 24.3108) construction
  line L5836 (66.7236, 24.3108) -> (66.8887, 24.2792) construction
  line L5837 (66.8887, 24.2792) -> (67.0208, 24.2532) construction
  line L5838 (67.0208, 24.2532) -> (67.1199, 24.2334) construction
  line L5839 (67.1199, 24.2334) -> (67.186, 24.22) construction
  line L5840 (67.186, 24.22) -> (67.2191, 24.2132) construction
  arc A149 (-5.5428, -59.1442) -> (-7.2806, -56.9737) centre (-7.5341, -58.9575) ccw
  spline S78 degree 5 poles (-52.5103, 31.1115) (-52.5368, 31.1272) (-52.5895, 31.1594) (-52.6672, 31.2097) (-52.7681, 31.2807) (-52.8906, 31.3748) (-53.0106, 31.4727) (-53.1289, 31.5729) (-53.2464, 31.6744) (-53.3634, 31.7767) (-53.4797, 31.88) (-53.5951, 31.9844) (-53.7094, 32.0903) (-53.8224, 32.1981) (-53.934, 32.3077) (-54.0444, 32.419) (-54.1537, 32.5316) (-54.2622, 32.6455) (-54.3698, 32.7603) (-54.4767, 32.876) (-54.5828, 32.9927) (-54.6881, 33.1105) (-54.7926, 33.2292) (-54.8961, 33.3491) (-54.9988, 33.47) (-55.1007, 33.5919) (-55.2017, 33.7148) (-55.302, 33.8386) (-55.4015, 33.9633) (-55.5003, 34.0888) (-55.5984, 34.2151) (-55.6957, 34.3423) (-55.7923, 34.4703) (-55.8881, 34.5991) (-55.9832, 34.7288) (-56.0776, 34.8592) (-56.1712, 34.9905) (-56.2642, 35.1224) (-56.3564, 35.2552) (-56.448, 35.3886) (-56.5388, 35.5228) (-56.629, 35.6577) (-56.7185, 35.7933) (-56.8073, 35.9295) (-56.8955, 36.0665) (-56.9829, 36.2042) (-57.0697, 36.3425) (-57.1558, 36.4815) (-57.2413, 36.6211) (-57.3261, 36.7614) (-57.4102, 36.9023) (-57.4937, 37.0438) (-57.5765, 37.186) (-57.6587, 37.3288) (-57.7403, 37.4721) (-57.8212, 37.6161) (-57.9014, 37.7607) (-57.981, 37.9058) (-58.06, 38.0515) (-58.1383, 38.1978) (-58.216, 38.3447) (-58.2931, 38.4921) (-58.3695, 38.6401) (-58.4453, 38.7886) (-58.5205, 38.9377) (-58.595, 39.0873) (-58.669, 39.2374) (-58.7423, 39.3881) (-58.8149, 39.5393) (-58.887, 39.6909) (-58.9584, 39.8431) (-59.0151, 39.9653) (-59.0573, 40.0572) (-59.0853, 40.1185) (-59.0993, 40.1492) knots 0 0 0 0 0 0 0.01428571 0.02857143 0.04285714 0.05714286 0.07142857 0.08571429 0.1 0.11428571 0.12857143 0.14285714 0.15714286 0.17142857 0.18571429 0.2 0.21428571 0.22857143 0.24285714 0.25714286 0.27142857 0.28571429 0.3 0.31428571 0.32857143 0.34285714 0.35714286 0.37142857 0.38571429 0.4 0.41428571 0.42857143 0.44285714 0.45714286 0.47142857 0.48571429 0.5 0.51428571 0.52857143 0.54285714 0.55714286 0.57142857 0.58571429 0.6 0.61428571 0.62857143 0.64285714 0.65714286 0.67142857 0.68571429 0.7 0.71428571 0.72857143 0.74285714 0.75714286 0.77142857 0.78571429 0.8 0.81428571 0.82857143 0.84285714 0.85714286 0.87142857 0.88571429 0.9 0.91428571 0.92857143 0.94285714 0.95714286 0.97142857 0.98571429 1 1 1 1 1 1
  line L5841 (-52.5103, 31.1115) -> (-52.5368, 31.1272) construction
  line L5842 (-52.5368, 31.1272) -> (-52.5895, 31.1594) construction
  line L5843 (-52.5895, 31.1594) -> (-52.6672, 31.2097) construction
  line L5844 (-52.6672, 31.2097) -> (-52.7681, 31.2807) construction
  line L5845 (-52.7681, 31.2807) -> (-52.8906, 31.3748) construction
  line L5846 (-52.8906, 31.3748) -> (-53.0106, 31.4727) construction
  line L5847 (-53.0106, 31.4727) -> (-53.1289, 31.5729) construction
  line L5848 (-53.1289, 31.5729) -> (-53.2464, 31.6744) construction
  line L5849 (-53.2464, 31.6744) -> (-53.3634, 31.7767) construction
  line L5850 (-53.3634, 31.7767) -> (-53.4797, 31.88) construction
  line L5851 (-53.4797, 31.88) -> (-53.5951, 31.9844) construction
  line L5852 (-53.5951, 31.9844) -> (-53.7094, 32.0903) construction
  line L5853 (-53.7094, 32.0903) -> (-53.8224, 32.1981) construction
  line L5854 (-53.8224, 32.1981) -> (-53.934, 32.3077) construction
  line L5855 (-53.934, 32.3077) -> (-54.0444, 32.419) construction
  line L5856 (-54.0444, 32.419) -> (-54.1537, 32.5316) construction
  line L5857 (-54.1537, 32.5316) -> (-54.2622, 32.6455) construction
  line L5858 (-54.2622, 32.6455) -> (-54.3698, 32.7603) construction
  line L5859 (-54.3698, 32.7603) -> (-54.4767, 32.876) construction
  line L5860 (-54.4767, 32.876) -> (-54.5828, 32.9927) construction
  line L5861 (-54.5828, 32.9927) -> (-54.6881, 33.1105) construction
  line L5862 (-54.6881, 33.1105) -> (-54.7926, 33.2292) construction
  line L5863 (-54.7926, 33.2292) -> (-54.8961, 33.3491) construction
  line L5864 (-54.8961, 33.3491) -> (-54.9988, 33.47) construction
  line L5865 (-54.9988, 33.47) -> (-55.1007, 33.5919) construction
  line L5866 (-55.1007, 33.5919) -> (-55.2017, 33.7148) construction
  line L5867 (-55.2017, 33.7148) -> (-55.302, 33.8386) construction
  line L5868 (-55.302, 33.8386) -> (-55.4015, 33.9633) construction
  line L5869 (-55.4015, 33.9633) -> (-55.5003, 34.0888) construction
  line L5870 (-55.5003, 34.0888) -> (-55.5984, 34.2151) construction
  line L5871 (-55.5984, 34.2151) -> (-55.6957, 34.3423) construction
  line L5872 (-55.6957, 34.3423) -> (-55.7923, 34.4703) construction
  line L5873 (-55.7923, 34.4703) -> (-55.8881, 34.5991) construction
  line L5874 (-55.8881, 34.5991) -> (-55.9832, 34.7288) construction
  line L5875 (-55.9832, 34.7288) -> (-56.0776, 34.8592) construction
  line L5876 (-56.0776, 34.8592) -> (-56.1712, 34.9905) construction
  line L5877 (-56.1712, 34.9905) -> (-56.2642, 35.1224) construction
  line L5878 (-56.2642, 35.1224) -> (-56.3564, 35.2552) construction
  line L5879 (-56.3564, 35.2552) -> (-56.448, 35.3886) construction
  line L5880 (-56.448, 35.3886) -> (-56.5388, 35.5228) construction
  line L5881 (-56.5388, 35.5228) -> (-56.629, 35.6577) construction
  line L5882 (-56.629, 35.6577) -> (-56.7185, 35.7933) construction
  line L5883 (-56.7185, 35.7933) -> (-56.8073, 35.9295) construction
  line L5884 (-56.8073, 35.9295) -> (-56.8955, 36.0665) construction
  line L5885 (-56.8955, 36.0665) -> (-56.9829, 36.2042) construction
  line L5886 (-56.9829, 36.2042) -> (-57.0697, 36.3425) construction
  line L5887 (-57.0697, 36.3425) -> (-57.1558, 36.4815) construction
  line L5888 (-57.1558, 36.4815) -> (-57.2413, 36.6211) construction
  line L5889 (-57.2413, 36.6211) -> (-57.3261, 36.7614) construction
  line L5890 (-57.3261, 36.7614) -> (-57.4102, 36.9023) construction
  line L5891 (-57.4102, 36.9023) -> (-57.4937, 37.0438) construction
  line L5892 (-57.4937, 37.0438) -> (-57.5765, 37.186) construction
  line L5893 (-57.5765, 37.186) -> (-57.6587, 37.3288) construction
  line L5894 (-57.6587, 37.3288) -> (-57.7403, 37.4721) construction
  line L5895 (-57.7403, 37.4721) -> (-57.8212, 37.6161) construction
  line L5896 (-57.8212, 37.6161) -> (-57.9014, 37.7607) construction
  line L5897 (-57.9014, 37.7607) -> (-57.981, 37.9058) construction
  line L5898 (-57.981, 37.9058) -> (-58.06, 38.0515) construction
  line L5899 (-58.06, 38.0515) -> (-58.1383, 38.1978) construction
  line L5900 (-58.1383, 38.1978) -> (-58.216, 38.3447) construction
  line L5901 (-58.216, 38.3447) -> (-58.2931, 38.4921) construction
  line L5902 (-58.2931, 38.4921) -> (-58.3695, 38.6401) construction
  line L5903 (-58.3695, 38.6401) -> (-58.4453, 38.7886) construction
  line L5904 (-58.4453, 38.7886) -> (-58.5205, 38.9377) construction
  line L5905 (-58.5205, 38.9377) -> (-58.595, 39.0873) construction
  line L5906 (-58.595, 39.0873) -> (-58.669, 39.2374) construction
  line L5907 (-58.669, 39.2374) -> (-58.7423, 39.3881) construction
  line L5908 (-58.7423, 39.3881) -> (-58.8149, 39.5393) construction
  line L5909 (-58.8149, 39.5393) -> (-58.887, 39.6909) construction
  line L5910 (-58.887, 39.6909) -> (-58.9584, 39.8431) construction
  line L5911 (-58.9584, 39.8431) -> (-59.0151, 39.9653) construction
  line L5912 (-59.0151, 39.9653) -> (-59.0573, 40.0572) construction
  line L5913 (-59.0573, 40.0572) -> (-59.0853, 40.1185) construction
  line L5914 (-59.0853, 40.1185) -> (-59.0993, 40.1492) construction
  arc A150 (40.1492, -59.0993) -> (43.8, -56.4469) centre (0, 0) ccw
  arc A151 (50.3721, -27.5982) -> (51.9354, -24.5301) centre (0, 0) ccw
  arc A152 (39.3784, -41.8132) -> (41.8132, -39.3784) centre (0, 0) ccw
  circle A153 centre (0, 0) radius 2.3
  line L5915 (-23.5481, 54.5366) -> (-24.1948, 56.0345)
  line L5916 (5.5428, 59.1442) -> (5.6951, 60.7685)
  line L5917 (54.5366, -23.5481) -> (56.0345, -24.1948)
  line L5918 (-5.5428, -59.1442) -> (-5.6951, -60.7685)
  line L5919 (-54.5366, -23.5481) -> (-56.0345, -24.1948)
  arc A154 (59.1442, -5.5428) -> (56.9737, -7.2806) centre (58.9575, -7.5341) ccw
  arc A155 (44.5906, -39.2483) -> (41.8132, -39.3784) centre (43.2692, -40.7496) ccw
  arc A156 (-51.9354, -24.5301) -> (-54.5366, -23.5481) centre (-53.7438, -25.3842) ccw
  arc A157 (-43.8, -56.4469) -> (-40.1492, -59.0993) centre (0, 0) ccw
  arc A158 (-2.2563, -71.4115) -> (2.2563, -71.4115) centre (0, 0) ccw
  spline S79 degree 5 poles (40.3263, 45.8153) (40.3467, 45.8385) (40.3868, 45.8854) (40.4451, 45.9573) (40.5192, 46.056) (40.6066, 46.1833) (40.6904, 46.3135) (40.772, 46.4454) (40.8524, 46.5782) (40.932, 46.7117) (41.0107, 46.8458) (41.0883, 46.9807) (41.1642, 47.1168) (41.2383, 47.2543) (41.3106, 47.393) (41.3813, 47.5329) (41.4504, 47.6738) (41.5184, 47.8156) (41.5853, 47.9581) (41.6512, 48.1012) (41.716, 48.245) (41.7798, 48.3895) (41.8424, 48.5347) (41.9039, 48.6807) (41.9642, 48.8274) (42.0234, 48.9749) (42.0815, 49.123) (42.1386, 49.2717) (42.1947, 49.421) (42.2499, 49.5709) (42.3041, 49.7214) (42.3574, 49.8724) (42.4097, 50.024) (42.461, 50.1761) (42.5114, 50.3288) (42.5608, 50.482) (42.6094, 50.6358) (42.657, 50.79) (42.7037, 50.9447) (42.7495, 51.0999) (42.7945, 51.2556) (42.8386, 51.4118) (42.8818, 51.5684) (42.9241, 51.7255) (42.9656, 51.883) (43.0063, 52.0409) (43.0461, 52.1993) (43.085, 52.3581) (43.1231, 52.5173) (43.1604, 52.6769) (43.1969, 52.8369) (43.2326, 52.9973) (43.2674, 53.1581) (43.3015, 53.3193) (43.3347, 53.4809) (43.3672, 53.6428) (43.3988, 53.8051) (43.4297, 53.9677) (43.4597, 54.1307) (43.489, 54.294) (43.5175, 54.4577) (43.5453, 54.6217) (43.5723, 54.7861) (43.5984, 54.9508) (43.6239, 55.1158) (43.6486, 55.2811) (43.6725, 55.4467) (43.6956, 55.6126) (43.718, 55.7789) (43.7397, 55.9454) (43.7606, 56.1122) (43.7767, 56.2459) (43.7885, 56.3463) (43.7962, 56.4133) (43.8, 56.4469) knots 0 0 0 0 0 0 0.01428571 0.02857143 0.04285714 0.05714286 0.07142857 0.08571429 0.1 0.11428571 0.12857143 0.14285714 0.15714286 0.17142857 0.18571429 0.2 0.21428571 0.22857143 0.24285714 0.25714286 0.27142857 0.28571429 0.3 0.31428571 0.32857143 0.34285714 0.35714286 0.37142857 0.38571429 0.4 0.41428571 0.42857143 0.44285714 0.45714286 0.47142857 0.48571429 0.5 0.51428571 0.52857143 0.54285714 0.55714286 0.57142857 0.58571429 0.6 0.61428571 0.62857143 0.64285714 0.65714286 0.67142857 0.68571429 0.7 0.71428571 0.72857143 0.74285714 0.75714286 0.77142857 0.78571429 0.8 0.81428571 0.82857143 0.84285714 0.85714286 0.87142857 0.88571429 0.9 0.91428571 0.92857143 0.94285714 0.95714286 0.97142857 0.98571429 1 1 1 1 1 1
  line L5920 (40.3263, 45.8153) -> (40.3467, 45.8385) construction
  line L5921 (40.3467, 45.8385) -> (40.3868, 45.8854) construction
  line L5922 (40.3868, 45.8854) -> (40.4451, 45.9573) construction
  line L5923 (40.4451, 45.9573) -> (40.5192, 46.056) construction
  line L5924 (40.5192, 46.056) -> (40.6066, 46.1833) construction
  line L5925 (40.6066, 46.1833) -> (40.6904, 46.3135) construction
  line L5926 (40.6904, 46.3135) -> (40.772, 46.4454) construction
  line L5927 (40.772, 46.4454) -> (40.8524, 46.5782) construction
  line L5928 (40.8524, 46.5782) -> (40.932, 46.7117) construction
  line L5929 (40.932, 46.7117) -> (41.0107, 46.8458) construction
  line L5930 (41.0107, 46.8458) -> (41.0883, 46.9807) construction
  line L5931 (41.0883, 46.9807) -> (41.1642, 47.1168) construction
  line L5932 (41.1642, 47.1168) -> (41.2383, 47.2543) construction
  line L5933 (41.2383, 47.2543) -> (41.3106, 47.393) construction
  line L5934 (41.3106, 47.393) -> (41.3813, 47.5329) construction
  line L5935 (41.3813, 47.5329) -> (41.4504, 47.6738) construction
  line L5936 (41.4504, 47.6738) -> (41.5184, 47.8156) construction
  line L5937 (41.5184, 47.8156) -> (41.5853, 47.9581) construction
  line L5938 (41.5853, 47.9581) -> (41.6512, 48.1012) construction
  line L5939 (41.6512, 48.1012) -> (41.716, 48.245) construction
  line L5940 (41.716, 48.245) -> (41.7798, 48.3895) construction
  line L5941 (41.7798, 48.3895) -> (41.8424, 48.5347) construction
  line L5942 (41.8424, 48.5347) -> (41.9039, 48.6807) construction
  line L5943 (41.9039, 48.6807) -> (41.9642, 48.8274) construction
  line L5944 (41.9642, 48.8274) -> (42.0234, 48.9749) construction
  line L5945 (42.0234, 48.9749) -> (42.0815, 49.123) construction
  line L5946 (42.0815, 49.123) -> (42.1386, 49.2717) construction
  line L5947 (42.1386, 49.2717) -> (42.1947, 49.421) construction
  line L5948 (42.1947, 49.421) -> (42.2499, 49.5709) construction
  line L5949 (42.2499, 49.5709) -> (42.3041, 49.7214) construction
  line L5950 (42.3041, 49.7214) -> (42.3574, 49.8724) construction
  line L5951 (42.3574, 49.8724) -> (42.4097, 50.024) construction
  line L5952 (42.4097, 50.024) -> (42.461, 50.1761) construction
  line L5953 (42.461, 50.1761) -> (42.5114, 50.3288) construction
  line L5954 (42.5114, 50.3288) -> (42.5608, 50.482) construction
  line L5955 (42.5608, 50.482) -> (42.6094, 50.6358) construction